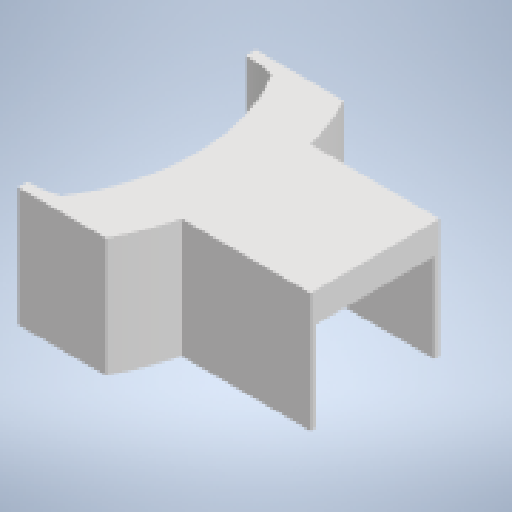
# Autodesk Inventor part: Chasis
Saved by Autodesk Inventor 2025.2 (Build 292293000, 293)
## iProperties
Created: 2025-04-24
Part Number: Chasis
Material: Genérico
Document SubType Name: Modeling
Designer: thmrc
Density: 1 g/cm^3
Appearance: Valor por defecto
Author: thmrc
Autodesk Inventor part; units mm, degrees
ref_plane "YZ Plane" through (0, 0, 0) normal (1, 0, 0) x (0, 1, 0)
ref_plane "XZ Plane" through (0, 0, 0) normal (0, 1, 0) x (-1, 0, 0)
ref_plane "XY Plane" through (0, 0, 0) normal (0, 0, 1) x (1, 0, 0)
sketch "Boceto2" plane through (0, 0, 0) normal (0, 1, 0) x (-1, 0, 0)
  line L0 (60, -60) -> (15.6267, -60)
  line L1 (15.6267, 60) -> (60, 60)
  arc A0 (45.1786, 52.9653) -> (45.1786, -52.9653) centre (130, 0) ccw
  arc A1 (45.1786, -52.9653) -> (60, -55) centre (60, 0) ccw
  arc A2 (60, 55) -> (45.1786, 52.9653) centre (60, 0) ccw
  line L2 (60, 60) -> (60, 55)
  line L3 (60, -55) -> (60, -60)
  line L4 (5, 32.5) -> (-60, 32.5)
  line L5 (5, -32.5) -> (-60, -32.5)
  line L6 (-60, -32.5) -> (-60, 32.5)
  arc A3 (15.6267, 60) -> (5, 32.5) centre (130, 0) ccw
  arc A4 (5, -32.5) -> (15.6267, -60) centre (130, 0) ccw
  line L7 (-60, 0) -> (60, 0) construction
  point P0 (0, 0)
  point P1 (30, 0)
  dimension "d8" = 200
  dimension "d13" = 65
  dimension "d17" = 65
  dimension "d18" = 65
  dimension "d19" = 30
  constraints: 16 end point, 11 point on circle, 5 centre point, 2 horizontal, 2 horizontal alignment, 1 coincident, 1 midpoint, 1 parallel, 1 vertical
  measures "d8" diameter of A0
  measures "d13" distance of L5.end L4.end
  measures "d17" distance of L4.start L4.end
  measures "d18" distance of L5.start L5.end
  measures "d19" distance of point (30, 0) L7.end
extrude "Extrusión1" add sketch "Boceto2" against normal blind 60
sketch "Boceto4" plane through (0, -60, 0) normal (0, -1, 0) x (1, 0, 0)
  line L0 (60, -32.5) -> (60, 32.5) projected
  line L1 (60, -30) -> (60, 30)
  arc A0 (-24.1699, -30) -> (-24.1699, 30) centre (-130, 0) ccw
  arc A1 (-45.1786, -52.9653) -> (-45.1786, 52.9653) centre (-130, 0) ccw projected
  line L2 (-24.1699, -30) -> (60, -30)
  line L3 (60, 30) -> (-24.1699, 30)
  point P0 (0, 0)
  point P1 (-40, 0)
  point P2 (-30, 0)
  dimension "d26" = 100
  dimension "d27" = 220
  dimension "d28" = 60
  constraints: 6 end point, 3 point on circle, 1 centre point, 1 horizontal, 1 horizontal alignment, 1 parallel, 1 perpendicular, 1 point on line
  measures "d26" distance of A0.centre point (-30, 0)
  measures "d27" diameter of A0
  measures "d28" distance between parallel lines of L3 L2
extrude "Extrusión2" cut sketch "Boceto4" against normal blind 45
sketch "Boceto5" plane through (-5, 0, 32.5) normal (0, 0, 1) x (1, 0, 0)
  line L0 (65, 0) -> (65, -60) projected
  line L1 (65, -60) -> (0, -60) projected
  line L2 (38.5, -26.2) -> (0, -26.2) construction
  line L3 (0, 0) -> (0, -60) projected
  arc A0 (26.666, -23.8432) -> (26.7187, -28.5748) centre (27.5, -26.2) ccw
  line L4 (36.4416, -20.3837) -> (26.666, -23.8432)
  line L5 (36.6445, -31.8401) -> (26.7187, -28.5748)
  line L6 (65, -29.7625) -> (43.25, -29.7625)
  line L7 (43.25, -22.2625) -> (65, -22.2625)
  line L8 (65, -22.2625) -> (65, -29.7625)
  arc A1 (36.6445, -31.8401) -> (43.25, -29.7625) centre (38.5, -26.2) ccw
  arc A2 (43.25, -22.2625) -> (36.4416, -20.3837) centre (38.5, -26.2) ccw
  circle A3 centre (18.5, -35.45) radius 1.625
  circle A4 centre (18.5, -16.95) radius 1.625
  point P0 (5, 0)
  point P1 (44.75, -26.2)
  dimension "d29" = 26.5
  dimension "d31" = 33.8
  dimension "d32" = 5
  dimension "d33" = 11
  dimension "d34" = 7.5
  dimension "d38" = 46.5
  dimension "d39" = 24.55
  dimension "d40" = 3.25
  constraints: 12 end point, 6 point on circle, 5 centre point, 4 tangent, 3 point on line, 2 horizontal, 1 parallel, 1 symmetric about line, 1 other
  measures "d29" distance from line of L0 L2.start
  measures "d31" distance from line of L1 L2.start
  measures "d32" diameter of A0
  measures "d33" distance of A0.centre L2.start
  measures "d34" distance between parallel lines of L7 L6
  measures "d38" distance from line of L0 A3.centre
  measures "d39" distance from line of L1 A3.centre
  measures "d40" diameter of A3
extrude "Extrusión3" cut sketch "Boceto5" against normal blind 65
sketch "Boceto7" plane through (0, -60, 0) normal (0, -1, 0) x (1, 0, 0)
  arc A0 (-24.1699, -30) -> (-24.1699, 30) centre (-130, 0) ccw projected
  line L0 (60, -30) -> (-24.1699, -30) projected
  line L1 (-24.1699, 30) -> (60, 30) projected
  line L2 (60, 30) -> (60, -30) projected
  point P0 (0, 0)
extrude "Extrusión4" add sketch "Boceto7" against normal blind 22
sketch "Boceto8" plane through (0, -60, 0) normal (0, -1, 0) x (1, 0, 0)
  line L0 (60, -30) -> (-24.1699, -30) projected
  arc A0 (-24.1699, -30) -> (-24.1699, 30) centre (-130, 0) ccw projected
  line L1 (-24.1699, 30) -> (60, 30) projected
  line L2 (60, -30) -> (60, 30)
  point P0 (0, 0)
  constraints: 2 end point, 1 perpendicular
extrude "Extrusión5" cut sketch "Boceto8" against normal blind 19.5
sketch "Boceto9" plane through (0, -40.5, 0) normal (0, -1, 0) x (1, 0, 0)
  line L0 (60, 8.5) -> (60, -8.5)
  arc A0 (-20.3289, -8.5) -> (-20.3289, 8.5) centre (-130, 0) ccw
  line L1 (60, 30) -> (60, -30) projected
  line L2 (60, -8.5) -> (-20.3289, -8.5)
  line L3 (60, 8.5) -> (-20.3289, 8.5)
  point P0 (0, 0)
  point P1 (60, -10)
  point P2 (60, 10)
  point P3 (-30, 0)
  dimension "d52" = 8.5
  dimension "d53" = 8.5
  constraints: 6 end point, 2 perpendicular, 2 point on circle, 2 point on line, 1 centre point, 1 coincident, 1 horizontal alignment
  measures "d52" distance from line of point (0, 0) L2
  measures "d53" distance from line of point (0, 0) L3
extrude "Extrusión6" cut sketch "Boceto9" against normal blind 2.5
sketch "Boceto10" plane through (0, -40.5, 0) normal (0, -1, 0) x (1, 0, 0)
  line L0 (55, 11.75) -> (8.5, 11.75) construction
  line L1 (8.5, 11.75) -> (8.5, -11.75) construction
  line L2 (8.5, -11.75) -> (55, -11.75) construction
  line L3 (55, -11.75) -> (55, 11.75) construction
  line L4 (60, 30) -> (60, 8.5) construction
  line L5 (-20.3289, 8.5) -> (60, 8.5) construction
  line L6 (58.25, 15) -> (51.75, 15)
  line L7 (51.75, 15) -> (51.75, 8.5)
  line L8 (51.75, 8.5) -> (58.25, 8.5)
  line L9 (58.25, 8.5) -> (58.25, 15)
  line L10 (58.25, 15) -> (51.75, 8.5) construction
  line L11 (51.75, 15) -> (58.25, 8.5) construction
  line L12 (60, -8.5) -> (-20.3289, -8.5) construction
  line L13 (58.25, -15) -> (51.75, -15)
  line L14 (51.75, -15) -> (51.75, -8.5)
  line L15 (51.75, -8.5) -> (58.25, -8.5)
  line L16 (58.25, -8.5) -> (58.25, -15)
  line L17 (58.25, -15) -> (51.75, -8.5) construction
  line L18 (51.75, -15) -> (58.25, -8.5) construction
  line L19 (5.25, -15) -> (11.75, -15)
  line L20 (11.75, -15) -> (11.75, -8.5)
  line L21 (11.75, -8.5) -> (5.25, -8.5)
  line L22 (5.25, -8.5) -> (5.25, -15)
  line L23 (5.25, -15) -> (11.75, -8.5) construction
  line L24 (11.75, -15) -> (5.25, -8.5) construction
  line L25 (11.75, 15) -> (5.25, 15)
  line L26 (5.25, 15) -> (5.25, 8.5)
  line L27 (5.25, 8.5) -> (11.75, 8.5)
  line L28 (11.75, 8.5) -> (11.75, 15)
  line L29 (11.75, 15) -> (5.25, 8.5) construction
  line L30 (5.25, 15) -> (11.75, 8.5) construction
  point P0 (0, 0)
  point P1 (8.5, 0)
  dimension "d50" = 46.5
  dimension "d51" = 23.5
  dimension "d54" = 5
  dimension "d55" = 6.5
  dimension "d56" = 6.5
  constraints: 56 end point, 10 parallel, 9 midpoint, 5 horizontal, 5 perpendicular, 5 point on line, 1 horizontal alignment
  measures "d50" distance of L0.start L0.end
  measures "d51" distance of L2.end L0.start
  measures "d54" distance between parallel lines of L4 L3
  measures "d55" distance of L8.end L7.end
  measures "d56" distance of L21.end L20.end
extrude "Extrusión7" add sketch "Boceto10" along normal blind 2.5
sketch "Boceto11" plane through (0, -43, 0) normal (0, -1, 0) x (1, 0, 0)
  line L0 (5.25, 8.5) -> (11.75, 8.5) construction
  line L1 (5.25, 8.5) -> (5.25, 11.75) construction
  line L2 (5.25, 8.5) -> (5.25, 15) construction
  line L3 (11.75, 8.5) -> (11.75, 15) construction
  line L4 (11.75, 11.75) -> (5.25, 11.75) construction
  line L5 (8.5, 11.75) -> (55, 11.75) construction
  line L6 (55, 11.75) -> (55, -11.75) construction
  line L7 (55, -11.75) -> (8.5, -11.75) construction
  line L8 (8.5, -11.75) -> (8.5, 11.75) construction
  circle A0 centre (8.5, 11.75) radius 1.625
  circle A1 centre (8.5, -11.75) radius 1.625
  circle A2 centre (55, 11.75) radius 1.625
  circle A3 centre (55, -11.75) radius 1.625
  point P0 (0, 0)
  dimension "d59" = 46.5
  dimension "d60" = 23.5
  dimension "d61" = 3.25
  dimension "d62" = 3.25
  dimension "d63" = 3.25
  dimension "d64" = 3.25
  constraints: 12 end point, 4 centre point, 4 coincident, 3 midpoint, 2 parallel, 2 perpendicular, 1 horizontal
  measures "d59" distance of L6.end L7.end
  measures "d60" distance of L5.end L6.end
  measures "d61" diameter of A0
  measures "d62" diameter of A1
  measures "d63" diameter of A2
  measures "d64" diameter of A3
extrude "Extrusión8" cut sketch "Boceto11" against normal blind 4
sketch "Boceto12" plane through (0, -60, 0) normal (0, -1, 0) x (1, 0, 0)
  arc A0 (-45.1786, -52.9653) -> (-45.1786, 52.9653) centre (-130, 0) ccw projected
  line L0 (-60, -60) -> (-15.6267, -60) projected
  line L1 (-23.3464, -55) -> (-34.7372, -55)
  arc A1 (-5, 32.5) -> (-15.6267, 60) centre (-130, 0) ccw projected
  line L2 (-23.3464, 55) -> (-34.7372, 55)
  arc A2 (-15.6267, -60) -> (-5, -32.5) centre (-130, 0) ccw projected
  arc A3 (-26.5894, 37.5) -> (-34.7372, 55) centre (-130, 0) ccw
  arc A4 (-34.7372, -55) -> (-26.5894, -37.5) centre (-130, 0) ccw
  arc A5 (-16.0099, 37.5) -> (-23.3464, 55) centre (-130, 0) ccw
  arc A6 (-23.3464, -55) -> (-16.0099, -37.5) centre (-130, 0) ccw
  line L3 (-16.0099, 37.5) -> (-26.5894, 37.5)
  line L4 (-16.0099, -37.5) -> (-26.5894, -37.5)
  point P0 (0, 0)
  constraints: 8 end point, 8 point on circle, 4 centre point, 2 coincident
extrude "Extrusión9" cut sketch "Boceto12" against normal blind 50
